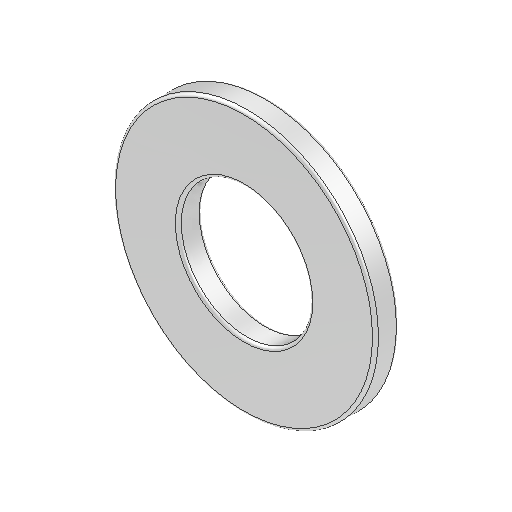
# Autodesk Inventor part: Arruela m4
Saved by Autodesk Inventor 2025 (Build 290162000, 162)
## iProperties
Created: 2024-12-11
Part Number: Arruela m4
Material: Aço inoxidável AISI 304
Document SubType Name: Modeling
Designer: November
Density: 8 g/cm^3
Appearance: Cromado - Acetinado
Author: November
Autodesk Inventor part; units mm, degrees
ref_plane "YZ Plane" through (0, 0, 0) normal (1, 0, 0) x (0, 1, 0)
ref_plane "XZ Plane" through (0, 0, 0) normal (0, 1, 0) x (-1, 0, 0)
ref_plane "XY Plane" through (0, 0, 0) normal (0, 0, 1) x (1, 0, 0)
sketch "Esboço1" plane through (0, 0, 0) normal (0, 0, 1) x (1, 0, 0)
  circle A0 centre (0, 0) radius 2.2
  circle A1 centre (0, 0) radius 4.4
  dimension "d0" = 4.4
  dimension "d1" = 8.8
  constraints: 2 centre point, 2 coincident
  measures "d0" diameter of A0
  measures "d1" diameter of A1
extrude "Extrusão1" add sketch "Esboço1" along normal blind 0.8
fillet "Arredondamento1" radius 0.1 1 edges at (-4.4, 0, 0.8)
fillet "Arredondamento2" radius 0.1 3 edges at (-2.2, 0, 0.8) (-4.4, 0, 0) (-2.2, 0, 0)
